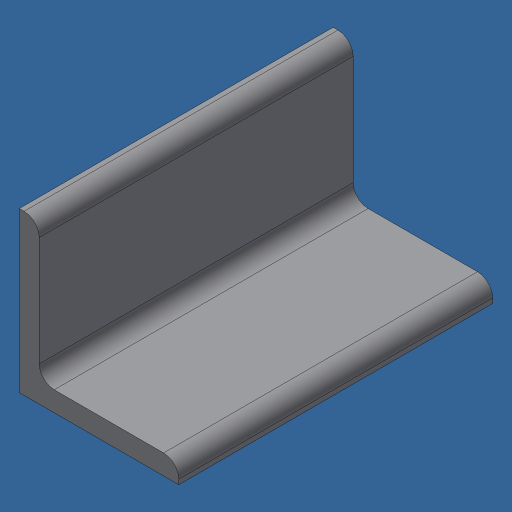
# Autodesk Inventor part: ANGLE IRON, 2 X 2 X 0.25 THK
Saved by Autodesk Inventor 2024.3 (Build 283343000, 343)
## iProperties
ILogicPurgeVersion: 2.2.20.20
OnSaveVersion: 2.2.20.20
Category: _
Manager: _
Part Number: ANGLE IRON, 2 X 2 X 0.25 THK
Checked By: 00
Engr Approved By: _
User Status: Work In Process
Material: Angle Iron
Description: ANGLE IRON, 2 X 2 X 0.25 THK
Document SubType Name: Modeling
Mfg Approved By: Stephen.Oerton
Designer: -
Mass: 471.371 g
Surface Area: 209.007 cm^2
Volume: 59.9709 cm^3
Density: 7.86 g/cm^3
Appearance: Grey (Light)
Created: 2023-11-08
CN_MASS: 0.47
CN_SERVICEABLE: _
CL_runCount: 0
FIRST_DESCRIPTION: _
SECOND_DESCRIPTION: _
THIRD_DESCRIPTION: _
ModelCat: Uncategorized
Subject: _
Author: -
Keywords: -
Revision Number: A
Autodesk Inventor part; units mm, degrees
ref_plane "YZ Plane" through (0, 0, 0) normal (1, 0, 0) x (0, 1, 0)
ref_plane "XZ Plane" through (0, 0, 0) normal (0, 1, 0) x (-1, 0, 0)
ref_plane "XY Plane" through (0, 0, 0) normal (0, 0, 1) x (1, 0, 0)
sketch "Sketch1" plane through (0, 0, 0) normal (0, 0, 1) x (1, 0, 0)
  line L0 (0, 0) -> (0, 50.8)
  line L1 (0, 50.8) -> (1.524, 50.8)
  line L2 (6.35, 45.974) -> (6.35, 11.1125)
  line L3 (0, 0) -> (50.8, 0)
  line L4 (50.8, 0) -> (50.8, 1.524)
  line L5 (45.974, 6.35) -> (11.1125, 6.35)
  arc A0 (6.35, 11.1125) -> (11.1125, 6.35) centre (11.1125, 11.1125) ccw
  arc A1 (6.35, 45.974) -> (1.524, 50.8) centre (1.524, 45.974) ccw
  arc A2 (50.8, 1.524) -> (45.974, 6.35) centre (45.974, 1.524) ccw
  dimension "thickness" = 6.35
  dimension "d3" = 6.35
  dimension "LegSize" = 50.8
  dimension "d5" = 50.8
  dimension "radius" = 4.7625
  dimension "d7" = 4.826
  dimension "d8" = 4.826
  constraints: 12 end point, 6 point on circle, 6 tangent, 4 parallel, 3 centre point, 1 coincident, 1 perpendicular, 1 vertical
  measures "thickness" distance between parallel lines of L2 L0
  measures "d3" distance between parallel lines of L5 L3
  measures "LegSize" distance of L0.start L0.end
  measures "d5" distance of L0.start L3.end
  measures "radius" radius of A0
  measures "d7" radius of A1
  measures "d8" radius of A2
extrude "2\" X 2\" X 1/4\"" add sketch "Sketch1" along normal mid plane 100
equation "\"d3\" = thickness"
equation "\"d5\" = LegSize"
